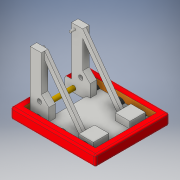
# Autodesk Inventor part: base
Saved by Autodesk Inventor 2016 (Build 200138000, 138)
## iProperties
Created: 2018-01-09
Part Number: base
Material: Generic
Document SubType Name: Modeling
Designer: New User
Density: 1 g/cm^3
Appearance: Default
Author: New User
Autodesk Inventor part; units mm, degrees
ref_plane "YZ Plane" through (0, 0, 0) normal (1, 0, 0) x (0, 1, 0)
ref_plane "XZ Plane" through (0, 0, 0) normal (0, 1, 0) x (-1, 0, 0)
ref_plane "XY Plane" through (0, 0, 0) normal (0, 0, 1) x (1, 0, 0)
sketch "Sketch1" plane through (0, 0, 0) normal (0, 1, 0) x (-1, 0, 0)
  line L0 (0, 0) -> (838.2, 0)
  line L1 (838.2, 0) -> (838.2, -711.2)
  line L2 (838.2, -711.2) -> (0, -711.2)
  line L3 (0, -711.2) -> (0, 0)
  line L4 (838.2, -152.4) -> (660.4, -152.4)
  line L5 (660.4, -152.4) -> (660.4, -558.8)
  line L6 (660.4, -558.8) -> (838.2, -558.8)
  line L7 (838.2, -558.8) -> (838.2, -152.4)
  dimension "d0" = 838.2
  dimension "d1" = 711.2
  dimension "d2" = 152.4
  dimension "d3" = 152.4
  dimension "d4" = 177.8
  constraints: 16 end point, 4 parallel, 2 horizontal, 2 perpendicular, 1 point on line
  measures "d0" distance of L1.end L2.end
  measures "d1" distance of L0.end L1.end
  measures "d2" distance between parallel lines of L2 L6
  measures "d3" distance between parallel lines of L0 L4
  measures "d4" distance between parallel lines of L1 L5
extrude "Extrusion1" add sketch "Sketch1" along normal blind 41.275 contours L0 L1 L4 L5 L6 L2 L3
sketch "Sketch2" plane through (-838.2, 0, 0) normal (0, 0, 1) x (1, 0, 0)
  line L0 (0, 0) -> (838.2, 0)
  line L1 (838.2, 0) -> (838.2, 127)
  line L2 (838.2, 127) -> (0, 127)
  line L3 (0, 127) -> (0, 0)
  dimension "d7" = 127
  dimension "d8" = 838.2
  constraints: 8 end point, 2 parallel, 1 horizontal, 1 perpendicular
  measures "d7" distance of L0.end L1.end
  measures "d8" distance of L1.end L2.end
extrude "Extrusion2" add sketch "Sketch2" along normal blind 76.2
sketch "Sketch3" plane through (0, 0, -711.2) normal (0, 0, -1) x (-1, 0, 0)
  line L0 (0, 127) -> (838.2, 127) projected
  line L1 (0, 127) -> (838.2, 127)
  line L2 (838.2, 127) -> (838.2, 0)
  line L3 (838.2, 0) -> (0, 0)
  line L4 (0, 0) -> (0, 127)
  constraints: 8 end point, 2 parallel, 1 horizontal, 1 perpendicular
extrude "Extrusion3" add sketch "Sketch3" along normal blind 76.2
sketch "Sketch4" plane through (-838.2, 0, -558.8) normal (-1, 0, 0) x (0, 0, 1)
  line L0 (-228.6, 127) -> (-228.6, 0) projected
  line L1 (-228.6, 0) -> (0, 0)
  line L2 (0, 0) -> (0, 127)
  line L3 (0, 127) -> (-228.6, 127)
  line L4 (-228.6, 127) -> (-228.6, 0)
  line L5 (635, 0) -> (635, 127) projected
  line L6 (635, 0) -> (406.4, 0)
  line L7 (406.4, 0) -> (406.4, 127)
  line L8 (406.4, 127) -> (635, 127)
  line L9 (635, 127) -> (635, 0)
  point P0 (558.8, 0)
  dimension "d13" = 228.6
  dimension "d14" = 228.6
  constraints: 16 end point, 4 parallel, 2 horizontal, 2 perpendicular
  measures "d13" distance of L2.end L3.end
  measures "d14" distance of L7.end L8.end
extrude "Extrusion4" add sketch "Sketch4" along normal blind 76.2
sketch "Sketch5" plane through (0, 41.275, 0) normal (1, 0, 0) x (0, 0, -1)
  line L0 (-76.2, -41.275) -> (787.4, -41.275)
  line L1 (787.4, -41.275) -> (787.4, 85.725)
  line L2 (787.4, 85.725) -> (-76.2, 85.725)
  line L3 (-76.2, 85.725) -> (-76.2, -41.275)
  constraints: 8 end point, 2 parallel, 1 horizontal, 1 perpendicular
extrude "Extrusion5" add sketch "Sketch5" along normal blind 76.2
fillet "Fillet1" radius 20.32 13 edges at (76.2, 127, -355.6) (76.2, 0, -355.6) (76.2, 63.5, -787.4) (-419.1, 127, -787.4) (-419.1, 0, -787.4) (-914.4, 127, -673.1) (-419.1, 127, 76.2) (-914.4, 127, -38.1) (-914.4, 0, -673.1) (-914.4, 0, -38.1) (-914.4, 63.5, 76.2) (76.2, 63.5, 76.2) (-419.1, 0, 76.2)
sketch "Sketch7" plane through (-838.2, 0, 0) normal (0, 0, -1) x (-1, 0, 0)
  line L0 (0, 41.275) -> (-838.2, 41.275) projected
  line L1 (0, 41.275) -> (-177.8, 41.275) projected
  line L2 (-894.08, 20.32) -> (55.88, 20.32) projected
  circle A0 centre (-127, 20.32) radius 63.5
  circle A1 centre (-419.1, 20.32) radius 63.5
  circle A2 centre (-673.6496, 20.32) radius 63.5
  point P0 (-838.2, 0)
  dimension "d28" = 127
  dimension "d29" = 127
  dimension "d30" = 127
  constraints: 3 centre point, 2 point on line, 1 midpoint
  measures "d28" diameter of A0
  measures "d29" diameter of A1
  measures "d30" diameter of A2
extrude "Extrusion7" add sketch "Sketch7" along normal blind 50.8 contours A0 L2 L0 | L0 A0 | A0 L2 | A1 L2 L0 | L0 A1 | A1 L2 | A2 L2 L0 | L0 A2 | A2 L2
sketch "Sketch6" plane through (0, 0, -711.2) normal (0, 0, 1) x (1, 0, 0)
  line L0 (-838.2, 41.275) -> (-660.4, 41.275) projected
  line L1 (-838.2, 41.275) -> (0, 41.275) projected
  line L2 (55.88, 127) -> (-894.08, 127) projected
  circle A0 centre (-711.2, 14.2491) radius 58.7603
  circle A1 centre (-419.1, 14.2491) radius 60.1045
  circle A2 centre (-163.5135, 14.2491) radius 57.477
  point P0 (0, 0)
  constraints: 3 centre point
extrude "Extrusion6" add sketch "Sketch6" along normal blind 50.8
sketch "Sketch8" plane through (0, 0, -660.4) normal (0, 0, 1) x (1, 0, 0)
  line L0 (55.88, 20.32) -> (-894.08, 20.32) projected
  line L1 (-245.7455, 119.7221) -> (-75.34, 119.7221)
  line L2 (-75.34, 119.7221) -> (-75.34, 20.32)
  line L3 (-75.34, 20.32) -> (-245.7455, 20.32)
  line L4 (-245.7455, 20.32) -> (-245.7455, 119.7221)
  point P0 (0, 0)
  constraints: 8 end point, 2 parallel, 1 horizontal, 1 perpendicular, 1 point on line
extrude "Extrusion8" add sketch "Sketch8" along normal blind 182.5625
sketch "Sketch9" plane through (-838.2, 0, -50.8) normal (0, 0, -1) x (-1, 0, 0)
  line L0 (-762.86, 119.7221) -> (-592.4545, 119.7221) projected
  line L1 (-762.86, 41.275) -> (-592.4545, 41.275) projected
  line L2 (-762.86, 119.7221) -> (-592.4545, 119.7221)
  line L3 (-592.4545, 119.7221) -> (-592.4545, 41.275)
  line L4 (-592.4545, 41.275) -> (-762.86, 41.275)
  line L5 (-762.86, 41.275) -> (-762.86, 119.7221)
  point P0 (-838.2, 0)
  constraints: 8 end point, 2 parallel, 1 horizontal, 1 perpendicular
extrude "Extrusion9" add sketch "Sketch9" along normal blind 182.5625
sketch "Sketch12" plane through (0, 41.275, 0) normal (0, 1, 0) x (1, 0, 0)
  line L0 (-838.2, 558.8) -> (-894.08, 558.8) projected
  line L1 (-838.2, 558.8) -> (-620.3934, 558.8)
  line L2 (-620.3934, 558.8) -> (-620.3934, 635)
  line L3 (-620.3934, 635) -> (-838.2, 635)
  line L4 (-838.2, 635) -> (-838.2, 558.8)
  line L5 (-838.2, 152.4) -> (-838.2, 0) projected
  line L6 (-838.2, 152.4) -> (-620.3934, 152.4)
  line L7 (-620.3934, 152.4) -> (-620.3934, 76.2)
  line L8 (-620.3934, 76.2) -> (-838.2, 76.2)
  line L9 (-838.2, 76.2) -> (-838.2, 152.4)
  point P0 (0, 0)
  dimension "d40" = 76.2
  dimension "d41" = 76.2
  constraints: 16 end point, 4 parallel, 2 horizontal, 2 perpendicular
  measures "d40" distance of L1.end L2.end
  measures "d41" distance of L6.end L7.end
extrude "Extrusion11" add sketch "Sketch12" along normal blind 233.3625
sketch "Sketch14" plane through (-620.3934, 41.275, -635) normal (0, 0, -1) x (-1, 0, 0)
  circle A0 centre (108.9033, 153.9875) radius 25.4
  point P0 (-620.3934, -41.275)
  dimension "d66" = 50.8
  constraints: 1 centre point
  measures "d66" diameter of A0
extrude "Extrusion12" cut sketch "Sketch14" against normal blind 623.8875
chamfer "Chamfer3" distance 87.3125 angle 45 2 edges at (-620.3934, 274.6375, -596.9) (-620.3934, 274.6375, -114.3)
sketch "Sketch21" plane through (-660.4, 0, -558.8) normal (0, 0, 1) x (1, 0, 0)
  circle A0 centre (-152.4, 49.0918) radius 25.4
  line L0 (-177.8, 127) -> (-177.8, 274.6375) projected
  point P0 (660.4, 0)
  point P1 (-177.8, 812.8)
  dimension "d77" = 50.8
  dimension "d80" = 25.4
  constraints: 1 centre point
  measures "d77" diameter of A0
  measures "d80" distance from line of L0 A0.centre
extrude "Extrusion19" add sketch "Sketch21" along normal blind 422.275
sketch "Sketch22" plane through (0, 274.6375, 0) normal (0, 1, 0) x (1, 0, 0)
  line L0 (-838.2, 635) -> (-838.2, 711.2) projected
  line L1 (-660.4, 558.8) -> (-894.08, 558.8) projected
  line L2 (-838.2, 635) -> (-707.7059, 635)
  line L3 (-707.7059, 635) -> (-707.7059, 558.8)
  line L4 (-707.7059, 558.8) -> (-838.2, 558.8)
  line L5 (-838.2, 558.8) -> (-838.2, 635)
  line L6 (-707.7059, 76.2) -> (-620.3934, 76.2) projected
  line L7 (-838.2, 152.4) -> (-838.2, 76.2) projected
  line L8 (-707.7059, 76.2) -> (-838.2, 76.2)
  line L9 (-838.2, 76.2) -> (-838.2, 152.4)
  line L10 (-838.2, 152.4) -> (-707.7059, 152.4)
  line L11 (-707.7059, 152.4) -> (-707.7059, 76.2)
  point P0 (0, 0)
  constraints: 16 end point, 4 parallel, 2 horizontal, 2 perpendicular, 1 point on line
extrude "Extrusion20" add sketch "Sketch22" along normal blind 422.275
sketch "Sketch25" plane through (-660.4, 0, -558.8) normal (0, 0, 1) x (1, 0, 0)
  line L0 (-47.3059, 274.6375) -> (-47.3059, 696.9125) projected
  line L1 (660.4, 127) -> (-177.8, 127) projected
  line L2 (-47.3059, 696.9125) -> (370.4445, 127)
  line L3 (325.4294, 94.0036) -> (-92.321, 663.9161)
  line L4 (-92.321, 663.9161) -> (-47.3059, 696.9125)
  line L5 (370.4445, 127) -> (424.5643, 53.1674)
  line L6 (424.5643, 53.1674) -> (379.5493, 20.171)
  line L7 (379.5493, 20.171) -> (325.4294, 94.0036)
  point P0 (660.4, 0)
  constraints: 12 end point, 2 parallel, 1 point on line
extrude "Extrusion21" add sketch "Sketch25" against normal blind 38.1
sketch "Sketch28" plane through (-660.4, 0, -152.4) normal (0, 0, -1) x (-1, 0, 0)
  line L0 (47.3059, 696.9125) -> (-414.6545, 66.6868) projected
  line L1 (47.3059, 696.9125) -> (92.321, 663.9161)
  line L2 (92.321, 663.9161) -> (-369.6395, 33.6904)
  line L3 (-369.6395, 33.6904) -> (-414.6545, 66.6868)
  line L4 (-414.6545, 66.6868) -> (47.3059, 696.9125)
  line L5 (-364.0799, 41.275) -> (47.3059, 602.5047) projected
  point P0 (-660.4, 0)
  constraints: 8 end point, 2 parallel, 2 perpendicular
extrude "Extrusion24" add sketch "Sketch28" against normal blind 38.1
sketch "Sketch29" plane through (-660.4, 0, -152.4) normal (0, 0, -1) x (-1, 0, 0)
  circle A0 centre (142.3019, 646.1125) radius 12.7
  line L0 (47.3059, 696.9125) -> (177.8, 696.9125) projected
  line L1 (47.3059, 274.6375) -> (47.3059, 696.9125) projected
  point P0 (-660.4, 0)
  dimension "d91" = 25.4
  dimension "d92" = 50.8
  dimension "d93" = 94.996
  constraints: 1 centre point
  measures "d91" diameter of A0
  measures "d92" distance from line of L0 A0.centre
  measures "d93" distance from line of L1 A0.centre
extrude "Extrusion25" add sketch "Sketch29" along normal blind 50.8
sketch "Sketch30" plane through (-660.4, 0, -558.8) normal (0, 0, 1) x (1, 0, 0)
  circle A0 centre (-142.5559, 646.1125) radius 12.7
  line L0 (-47.3059, 274.6375) -> (-47.3059, 696.9125) projected
  line L1 (-177.8, 696.9125) -> (-47.3059, 696.9125) projected
  point P0 (660.4, 0)
  dimension "d96" = 25.4
  dimension "d97" = 95.25
  dimension "d98" = 50.8
  constraints: 1 centre point
  measures "d96" diameter of A0
  measures "d97" distance from line of L0 A0.centre
  measures "d98" distance from line of L1 A0.centre
extrude "Extrusion26" add sketch "Sketch30" along normal blind 50.8
body "Solid1"
